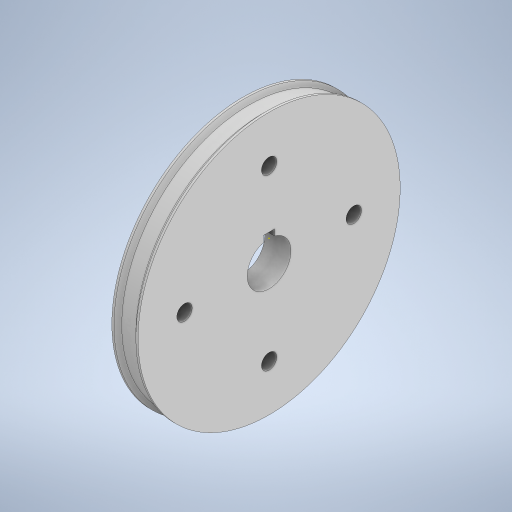
# Autodesk Inventor part: Polea_EjercicioClase
Saved by Autodesk Inventor 2024 (Build 280153000, 153)
## iProperties
Created: 2024-02-06
Part Number: Polea_EjercicioClase
Material: Genérico
Document SubType Name: Modeling
Designer: pazjo
Density: 1 g/cm^3
Appearance: Valor por defecto
Author: pazjo
Autodesk Inventor part; units mm, degrees
ref_plane "YZ Plane" through (0, 0, 0) normal (1, 0, 0) x (0, 1, 0)
ref_plane "XZ Plane" through (0, 0, 0) normal (0, 1, 0) x (-1, 0, 0)
ref_plane "XY Plane" through (0, 0, 0) normal (0, 0, 1) x (1, 0, 0)
sketch "Boceto1" plane through (0, 0, 0) normal (0, 0, 1) x (1, 0, 0)
  line L0 (0, 0) -> (100, 0)
  line L1 (100, 0) -> (100, 500)
  line L2 (0, 500) -> (0, 0)
  line L3 (0, 500) -> (17.6777, 482.3223)
  line L4 (100, 500) -> (82.3223, 482.3223)
  line L5 (17.6777, 482.3223) -> (82.3223, 482.3223)
  line L6 (50, -100) -> (-150, -100)
  constraints: 14 end point, 3 horizontal, 1 parallel, 1 perpendicular
revolve "Revolución1" add sketch "Boceto1" angle 360 about axis through (50, -100, 0) along (-1, 0, 0)
sketch "Boceto2" plane through (100, -100, 0) normal (1, 0, 0) x (0, 0, -1)
  circle A0 centre (0, 0) radius 600 construction
  circle A1 centre (-387.4756, 0) radius 35
  circle A2 centre (0, 0) radius 100 construction
  circle A3 centre (0, -387.4756) radius 35
  circle A4 centre (387.4756, 0) radius 35
  circle A5 centre (0, 387.4756) radius 35
  point P0 (0, 100)
  dimension "d13" = 360
  constraints: 5 centre point, 1 coincident, 9 other
extrude "Extrusión1" cut sketch "Boceto2" against normal through all
thicken "Engrosado1" operation add thickness 10 both sides no extend neighbours no toward (1, 0, 0) faces at (100, -375.8968, 274.6836)
thicken "Engrosado2" operation add thickness 10 both sides no extend neighbours no toward (-1, 0, 0) faces at (0, -375.8968, 274.6836)
sketch "Boceto3" plane through (110, -100, 0) normal (1, 0, 0) x (0, 0, -1)
  line L0 (25, 96.8246) -> (25, 125)
  line L1 (25, 125) -> (-25, 125)
  line L2 (-25, 125) -> (-25, 96.8246)
  line L3 (0, 100) -> (25, 125) construction
  line L4 (0, 100) -> (-25, 125) construction
  arc A0 (25, 96.8246) -> (-25, 96.8246) centre (0, 0) ccw
  point P0 (0, 100)
  constraints: 10 end point, 2 point on circle, 2 point on line, 1 centre point, 1 parallel
extrude "Extrusión2" cut sketch "Boceto3" against normal blind 120
sketch "Boceto4" plane through (110, -100, 0) normal (1, 0, 0) x (0, 0, -1)
  point P0 (0, 100)
